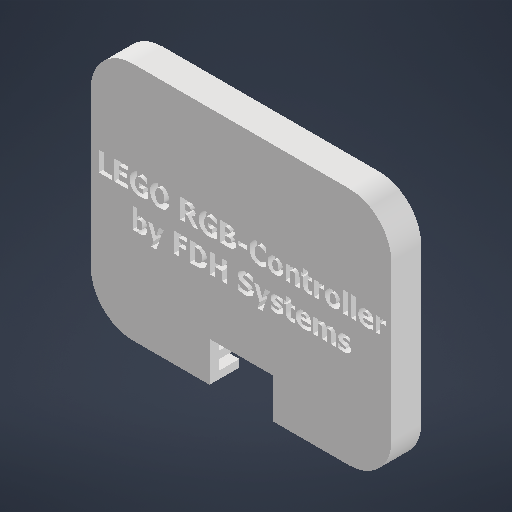
# Autodesk Inventor part: TopShell
Saved by Autodesk Inventor 2026.2 (Build 302298000, 298)
## iProperties
Created: 2026-04-30
Part Number: TopShell
Material: Generic
Document SubType Name: Modeling
Designer: FromDarkHell
Density: 1 g/cm^3
Appearance: Default
Author: FromDarkHell
Autodesk Inventor part; units mm, degrees
ref_plane "YZ Plane" through (0, 0, 0) normal (1, 0, 0) x (0, 1, 0)
ref_plane "XZ Plane" through (0, 0, 0) normal (0, 1, 0) x (-1, 0, 0)
ref_plane "XY Plane" through (0, 0, 0) normal (0, 0, 1) x (1, 0, 0)
sketch "Sketch4" plane through (0, 0, 0) normal (0, 0, 1) x (1, 0, 0)
  arc A0 (29.04, -4) -> (22.04, 3) centre (22.04, -4) ccw projected
  line L0 (29.04, -4) -> (29.04, -35.25) projected
  arc A1 (22.04, -42.25) -> (29.04, -35.25) centre (22.04, -35.25) ccw projected
  line L1 (22.04, -42.25) -> (-21.46, -42.25) projected
  arc A2 (-28.46, -35.25) -> (-21.46, -42.25) centre (-21.46, -35.25) ccw projected
  line L2 (-28.46, -35.25) -> (-28.46, -4) projected
  arc A3 (-21.46, 3) -> (-28.46, -4) centre (-21.46, -4) ccw projected
  line L3 (-21.46, 3) -> (22.04, 3) projected
  line L4 (-26.46, -35.25) -> (-26.46, -4) projected
  arc A4 (-21.46, 1) -> (-26.46, -4) centre (-21.46, -4) ccw projected
  line L5 (-21.46, 1) -> (22.04, 1) projected
  arc A5 (27.04, -4) -> (22.04, 1) centre (22.04, -4) ccw projected
  line L6 (27.04, -4) -> (27.04, -35.25) projected
  arc A6 (22.04, -40.25) -> (27.04, -35.25) centre (22.04, -35.25) ccw projected
  line L7 (22.04, -40.25) -> (-21.46, -40.25) projected
  arc A7 (-26.46, -35.25) -> (-21.46, -40.25) centre (-21.46, -35.25) ccw projected
  line L8 (-29.96, -4) -> (-29.96, -35.25)
  arc A8 (-29.96, -35.25) -> (-21.46, -43.75) centre (-21.46, -35.25) ccw
  line L9 (-21.46, -43.75) -> (22.04, -43.75)
  arc A9 (22.04, -43.75) -> (30.54, -35.25) centre (22.04, -35.25) ccw
  line L10 (30.54, -35.25) -> (30.54, -4)
  arc A10 (30.54, -4) -> (22.04, 4.5) centre (22.04, -4) ccw
  line L11 (22.04, 4.5) -> (-21.46, 4.5)
  arc A11 (-21.46, 4.5) -> (-29.96, -4) centre (-21.46, -4) ccw
  line L12 (-24.96, -4) -> (-24.96, -35.25)
  arc A12 (-24.96, -35.25) -> (-21.46, -38.75) centre (-21.46, -35.25) ccw
  line L13 (-21.46, -38.75) -> (22.04, -38.75)
  arc A13 (22.04, -38.75) -> (25.54, -35.25) centre (22.04, -35.25) ccw
  line L14 (25.54, -35.25) -> (25.54, -4)
  arc A14 (25.54, -4) -> (22.04, -0.5) centre (22.04, -4) ccw
  line L15 (22.04, -0.5) -> (-21.46, -0.5)
  arc A15 (-21.46, -0.5) -> (-24.96, -4) centre (-21.46, -4) ccw
  point P0 (0, 0)
  dimension "d18" = 1.5
  dimension "d19" = 1.5
  constraints: 16 end point, 16 point on circle, 8 centre point, 14 other
  measures "d18" radial gap between concentric circles of A3 A11
  measures "d19" distance between parallel lines of L4 L12
extrude "Extrusion5" add sketch "Sketch4" along normal blind 4
sketch "Sketch5" plane through (0, 0, 4) normal (0, 0, 1) x (1, 0, 0)
  arc A0 (-29.96, -35.25) -> (-21.46, -43.75) centre (-21.46, -35.25) ccw projected
  line L0 (-21.46, -43.75) -> (22.04, -43.75) projected
  arc A1 (22.04, -43.75) -> (30.54, -35.25) centre (22.04, -35.25) ccw projected
  line L1 (30.54, -35.25) -> (30.54, -4) projected
  arc A2 (30.54, -4) -> (22.04, 4.5) centre (22.04, -4) ccw projected
  line L2 (22.04, 4.5) -> (-21.46, 4.5) projected
  arc A3 (-21.46, 4.5) -> (-29.96, -4) centre (-21.46, -4) ccw projected
  line L3 (-29.96, -4) -> (-29.96, -35.25) projected
  line L4 (22.04, -42.25) -> (-21.46, -42.25) projected
  arc A4 (-28.46, -35.25) -> (-21.46, -42.25) centre (-21.46, -35.25) ccw projected
  line L5 (-28.46, -35.25) -> (-28.46, -4) projected
  arc A5 (-21.46, 3) -> (-28.46, -4) centre (-21.46, -4) ccw projected
  line L6 (-21.46, 3) -> (22.04, 3) projected
  arc A6 (29.04, -4) -> (22.04, 3) centre (22.04, -4) ccw projected
  line L7 (29.04, -4) -> (29.04, -35.25) projected
  arc A7 (22.04, -42.25) -> (29.04, -35.25) centre (22.04, -35.25) ccw projected
  point P0 (0, 0)
extrude "Extrusion6" add sketch "Sketch5" along normal blind 2 contours L3 A3 L2 A2 L1 A1 L0 A0 | L4 A4 L5 A5 L6 A6 L7 A7
sketch "Sketch6" plane through (0, 0, 6) normal (0, 0, 1) x (1, 0, 0)
  line L0 (-21.46, -43.75) -> (22.04, -43.75) projected
  arc A0 (22.04, -43.75) -> (30.54, -35.25) centre (22.04, -35.25) ccw projected
  line L1 (30.54, -35.25) -> (30.54, -4) projected
  arc A1 (30.54, -4) -> (22.04, 4.5) centre (22.04, -4) ccw projected
  line L2 (22.04, 4.5) -> (-21.46, 4.5) projected
  arc A2 (-21.46, 4.5) -> (-29.96, -4) centre (-21.46, -4) ccw projected
  line L3 (-29.96, -4) -> (-29.96, -35.25) projected
  arc A3 (-29.96, -35.25) -> (-21.46, -43.75) centre (-21.46, -35.25) ccw projected
  line L4 (-29.96, -19.625) -> (30.54, -19.625) construction
  line L5 (0.29, 4.5) -> (0.29, -43.75) construction
  line L6 (-28.8096, -14.0054) -> (29.3896, -14.0054) construction
  line L7 (29.3896, -14.0054) -> (29.3896, -25.2446) construction
  line L8 (29.3896, -25.2446) -> (-28.8096, -25.2446) construction
  line L9 (-28.8096, -25.2446) -> (-28.8096, -14.0054) construction
  line L10 (-25.7163, -17.8739) -> (-28.3759, -17.8739)
  line L11 (-28.3759, -17.8739) -> (-28.3759, -13.8861)
  line L12 (-28.3759, -13.8861) -> (-27.3741, -13.8861)
  line L13 (-27.3741, -13.8861) -> (-27.3741, -17.1144)
  line L14 (-27.3741, -17.1144) -> (-25.7163, -17.1144)
  line L15 (-25.7163, -17.1144) -> (-25.7163, -17.8739)
  line L16 (-25.2381, -17.8739) -> (-25.2381, -13.8861)
  line L17 (-25.2381, -13.8861) -> (-22.5429, -13.8861)
  line L18 (-22.5429, -13.8861) -> (-22.5429, -14.6455)
  line L19 (-22.5429, -14.6455) -> (-24.2427, -14.6455)
  line L20 (-24.2427, -14.6455) -> (-24.2427, -15.3468)
  line L21 (-24.2427, -15.3468) -> (-22.6754, -15.3468)
  line L22 (-22.6754, -15.3468) -> (-22.6754, -16.1062)
  line L23 (-22.6754, -16.1062) -> (-24.2427, -16.1062)
  line L24 (-24.2427, -16.1062) -> (-24.2427, -17.1144)
  line L25 (-24.2427, -17.1144) -> (-22.5429, -17.1144)
  line L26 (-22.5429, -17.1144) -> (-22.5429, -17.8739)
  line L27 (-22.5429, -17.8739) -> (-25.2381, -17.8739)
  spline S0 degree 2 poles (-18.5357, -17.6477) (-18.7975, -17.7543) (-19.6345, -17.9579) (-20.0416, -17.9579) knots 0 0 0 1 2 2 2
  spline S1 degree 2 poles (-20.0416, -17.9579) (-20.982, -17.9579) (-22.0969, -16.8721) (-22.0969, -15.8767) knots 0 0 0 1 2 2 2
  spline S2 degree 2 poles (-22.0969, -15.8767) (-22.0969, -14.9396) (-20.982, -13.8085) (-20.0126, -13.8085) knots 0 0 0 1 2 2 2
  spline S3 degree 2 poles (-20.0126, -13.8085) (-19.5117, -13.8085) (-18.8847, -13.9992) (-18.5519, -14.1608) knots 0 0 0 1 2 2 2
  line L28 (-18.5519, -14.1608) -> (-18.5519, -15.0979)
  line L29 (-18.5519, -15.0979) -> (-18.6424, -15.0979)
  spline S4 degree 2 poles (-18.6424, -15.0979) (-18.7134, -15.043) (-18.9849, -14.8329) (-19.1142, -14.7618) knots 0 0 0 1 2 2 2
  spline S5 degree 2 poles (-19.1142, -14.7618) (-19.2628, -14.6746) (-19.6571, -14.5518) (-19.8768, -14.5518) knots 0 0 0 1 2 2 2
  spline S6 degree 2 poles (-19.8768, -14.5518) (-20.1321, -14.5518) (-20.5555, -14.7134) (-20.7203, -14.8782) knots 0 0 0 1 2 2 2
  spline S7 degree 2 poles (-20.7203, -14.8782) (-20.8786, -15.0398) (-21.0628, -15.5342) (-21.0628, -15.8606) knots 0 0 0 1 2 2 2
  spline S8 degree 2 poles (-21.0628, -15.8606) (-21.0628, -16.5586) (-20.3616, -17.2243) (-19.7573, -17.2243) knots 0 0 0 1 2 2 2
  spline S9 degree 2 poles (-19.7573, -17.2243) (-19.7023, -17.2243) (-19.5601, -17.2179) (-19.5052, -17.2146) knots 0 0 0 1 2 2 2
  line L30 (-19.5052, -17.2146) -> (-19.5052, -16.4293)
  line L31 (-19.5052, -16.4293) -> (-20.2775, -16.4293)
  line L32 (-20.2775, -16.4293) -> (-20.2775, -15.6828)
  line L33 (-20.2775, -15.6828) -> (-18.5357, -15.6828)
  line L34 (-18.5357, -15.6828) -> (-18.5357, -17.6477)
  spline S10 degree 2 poles (-14.1504, -15.88) (-14.1504, -16.8495) (-15.1845, -17.9579) (-16.0829, -17.9579) knots 0 0 0 1 2 2 2
  spline S11 degree 2 poles (-16.0829, -17.9579) (-16.9845, -17.9579) (-18.0122, -16.8365) (-18.0122, -15.88) knots 0 0 0 1 2 2 2
  spline S12 degree 2 poles (-18.0122, -15.88) (-18.0122, -14.9202) (-16.9845, -13.8021) (-16.0829, -13.8021) knots 0 0 0 1 2 2 2
  spline S13 degree 2 poles (-16.0829, -13.8021) (-15.1845, -13.8021) (-14.1504, -14.9137) (-14.1504, -15.88) knots 0 0 0 1 2 2 2
  spline S14 degree 2 poles (-15.1845, -15.88) (-15.1845, -15.5213) (-15.33, -15.0204) (-15.456, -14.862) knots 0 0 0 1 2 2 2
  spline S15 degree 2 poles (-15.456, -14.862) (-15.582, -14.6972) (-15.9052, -14.555) (-16.0797, -14.555) knots 0 0 0 1 2 2 2
  spline S16 degree 2 poles (-16.0797, -14.555) (-16.2639, -14.555) (-16.5644, -14.6875) (-16.7034, -14.8556) knots 0 0 0 1 2 2 2
  spline S17 degree 2 poles (-16.7034, -14.8556) (-16.8262, -15.0107) (-16.9781, -15.5245) (-16.9781, -15.88) knots 0 0 0 1 2 2 2
  spline S18 degree 2 poles (-16.9781, -15.88) (-16.9781, -16.2484) (-16.8327, -16.7331) (-16.7066, -16.8979) knots 0 0 0 1 2 2 2
  spline S19 degree 2 poles (-16.7066, -16.8979) (-16.5806, -17.0627) (-16.2542, -17.2049) (-16.0797, -17.2049) knots 0 0 0 1 2 2 2
  spline S20 degree 2 poles (-16.0797, -17.2049) (-15.902, -17.2049) (-15.5723, -17.053) (-15.4528, -16.8915) knots 0 0 0 1 2 2 2
  spline S21 degree 2 poles (-15.4528, -16.8915) (-15.3235, -16.717) (-15.1845, -16.2548) (-15.1845, -15.88) knots 0 0 0 1 2 2 2
  line L35 (-8.2657, -17.8739) -> (-9.484, -17.8739)
  line L36 (-9.484, -17.8739) -> (-10.5924, -16.41)
  line L37 (-10.5924, -16.41) -> (-10.9544, -16.41)
  line L38 (-10.9544, -16.41) -> (-10.9544, -17.8739)
  line L39 (-10.9544, -17.8739) -> (-11.9497, -17.8739)
  line L40 (-11.9497, -17.8739) -> (-11.9497, -13.8861)
  line L41 (-11.9497, -13.8861) -> (-10.3468, -13.8861)
  spline S22 degree 2 poles (-10.3468, -13.8861) (-10.014, -13.8861) (-9.5228, -13.9701) (-9.3127, -14.0994) knots 0 0 0 1 2 2 2
  spline S23 degree 2 poles (-9.3127, -14.0994) (-9.0994, -14.2351) (-8.8474, -14.6584) (-8.8474, -14.9816) knots 0 0 0 1 2 2 2
  spline S24 degree 2 poles (-8.8474, -14.9816) (-8.8474, -15.4372) (-9.261, -16.0092) (-9.6068, -16.1773) knots 0 0 0 1 2 2 2
  line L42 (-9.6068, -16.1773) -> (-8.2657, -17.8739)
  spline S25 degree 2 poles (-9.875, -15.1076) (-9.875, -14.9557) (-9.9913, -14.7392) (-10.1238, -14.6811) knots 0 0 0 1 2 2 2
  spline S26 degree 2 poles (-10.1238, -14.6811) (-10.2176, -14.6423) (-10.447, -14.6197) (-10.6183, -14.6197) knots 0 0 0 1 2 2 2
  line L43 (-10.6183, -14.6197) -> (-10.9544, -14.6197)
  line L44 (-10.9544, -14.6197) -> (-10.9544, -15.6925)
  line L45 (-10.9544, -15.6925) -> (-10.6668, -15.6925)
  spline S27 degree 2 poles (-10.6668, -15.6925) (-10.4599, -15.6925) (-10.1659, -15.6408) (-10.0657, -15.56) knots 0 0 0 1 2 2 2
  spline S28 degree 2 poles (-10.0657, -15.56) (-9.9687, -15.4825) (-9.875, -15.2757) (-9.875, -15.1076) knots 0 0 0 1 2 2 2
  spline S29 degree 2 poles (-4.6398, -17.6477) (-4.9016, -17.7543) (-5.7386, -17.9579) (-6.1457, -17.9579) knots 0 0 0 1 2 2 2
  spline S30 degree 2 poles (-6.1457, -17.9579) (-7.0861, -17.9579) (-8.201, -16.8721) (-8.201, -15.8767) knots 0 0 0 1 2 2 2
  spline S31 degree 2 poles (-8.201, -15.8767) (-8.201, -14.9396) (-7.0861, -13.8085) (-6.1167, -13.8085) knots 0 0 0 1 2 2 2
  spline S32 degree 2 poles (-6.1167, -13.8085) (-5.6158, -13.8085) (-4.9888, -13.9992) (-4.656, -14.1608) knots 0 0 0 1 2 2 2
  line L46 (-4.656, -14.1608) -> (-4.656, -15.0979)
  line L47 (-4.656, -15.0979) -> (-4.7465, -15.0979)
  spline S33 degree 2 poles (-4.7465, -15.0979) (-4.8176, -15.043) (-5.089, -14.8329) (-5.2183, -14.7618) knots 0 0 0 1 2 2 2
  spline S34 degree 2 poles (-5.2183, -14.7618) (-5.3669, -14.6746) (-5.7612, -14.5518) (-5.9809, -14.5518) knots 0 0 0 1 2 2 2
  spline S35 degree 2 poles (-5.9809, -14.5518) (-6.2362, -14.5518) (-6.6596, -14.7134) (-6.8244, -14.8782) knots 0 0 0 1 2 2 2
  spline S36 degree 2 poles (-6.8244, -14.8782) (-6.9827, -15.0398) (-7.1669, -15.5342) (-7.1669, -15.8606) knots 0 0 0 1 2 2 2
  spline S37 degree 2 poles (-7.1669, -15.8606) (-7.1669, -16.5586) (-6.4657, -17.2243) (-5.8614, -17.2243) knots 0 0 0 1 2 2 2
  spline S38 degree 2 poles (-5.8614, -17.2243) (-5.8064, -17.2243) (-5.6642, -17.2179) (-5.6093, -17.2146) knots 0 0 0 1 2 2 2
  line L48 (-5.6093, -17.2146) -> (-5.6093, -16.4293)
  line L49 (-5.6093, -16.4293) -> (-6.3816, -16.4293)
  line L50 (-6.3816, -16.4293) -> (-6.3816, -15.6828)
  line L51 (-6.3816, -15.6828) -> (-4.6398, -15.6828)
  line L52 (-4.6398, -15.6828) -> (-4.6398, -17.6477)
  spline S39 degree 2 poles (-0.6973, -16.6523) (-0.6973, -16.9496) (-0.9235, -17.3988) (-1.1109, -17.5475) knots 0 0 0 1 2 2 2
  spline S40 degree 2 poles (-1.1109, -17.5475) (-1.3371, -17.7252) (-1.8736, -17.8739) (-2.2904, -17.8739) knots 0 0 0 1 2 2 2
  line L53 (-2.2904, -17.8739) -> (-3.8836, -17.8739)
  line L54 (-3.8836, -17.8739) -> (-3.8836, -13.8861)
  line L55 (-3.8836, -13.8861) -> (-2.4779, -13.8861)
  spline S41 degree 2 poles (-2.4779, -13.8861) (-2.0384, -13.8861) (-1.5859, -13.9539) (-1.3888, -14.0606) knots 0 0 0 1 2 2 2
  spline S42 degree 2 poles (-1.3888, -14.0606) (-1.1723, -14.1737) (-0.9622, -14.5615) (-0.9622, -14.8135) knots 0 0 0 1 2 2 2
  spline S43 degree 2 poles (-0.9622, -14.8135) (-0.9622, -15.1044) (-1.2531, -15.56) (-1.5116, -15.6667) knots 0 0 0 1 2 2 2
  line L56 (-1.5116, -15.6667) -> (-1.5116, -15.6861)
  spline S44 degree 2 poles (-1.5116, -15.6861) (-1.14, -15.7636) (-0.6973, -16.2451) (-0.6973, -16.6523) knots 0 0 0 1 2 2 2
  spline S45 degree 2 poles (-1.7314, -16.6362) (-1.7314, -16.4487) (-1.88, -16.2387) (-2.0287, -16.1837) knots 0 0 0 1 2 2 2
  spline S46 degree 2 poles (-2.0287, -16.1837) (-2.1192, -16.1482) (-2.4391, -16.1417) (-2.7041, -16.1417) knots 0 0 0 1 2 2 2
  line L57 (-2.7041, -16.1417) -> (-2.8883, -16.1417)
  line L58 (-2.8883, -16.1417) -> (-2.8883, -17.1468)
  line L59 (-2.8883, -17.1468) -> (-2.8333, -17.1468)
  spline S47 degree 2 poles (-2.8333, -17.1468) (-2.4456, -17.1468) (-2.1482, -17.1371) (-1.9931, -17.0692) knots 0 0 0 1 2 2 2
  spline S48 degree 2 poles (-1.9931, -17.0692) (-1.8574, -17.0078) (-1.7314, -16.7816) (-1.7314, -16.6362) knots 0 0 0 1 2 2 2
  spline S49 degree 2 poles (-1.9802, -15.0107) (-1.9802, -14.9137) (-2.0804, -14.7101) (-2.1838, -14.6649) knots 0 0 0 1 2 2 2
  spline S50 degree 2 poles (-2.1838, -14.6649) (-2.2807, -14.6197) (-2.5522, -14.6132) (-2.8204, -14.6132) knots 0 0 0 1 2 2 2
  line L60 (-2.8204, -14.6132) -> (-2.8883, -14.6132)
  line L61 (-2.8883, -14.6132) -> (-2.8883, -15.4599)
  line L62 (-2.8883, -15.4599) -> (-2.7623, -15.4599)
  spline S51 degree 2 poles (-2.7623, -15.4599) (-2.507, -15.4599) (-2.3001, -15.4502) (-2.1903, -15.3985) knots 0 0 0 1 2 2 2
  spline S52 degree 2 poles (-2.1903, -15.3985) (-2.0707, -15.3403) (-1.9802, -15.1432) (-1.9802, -15.0107) knots 0 0 0 1 2 2 2
  line L63 (1.5326, -16.4843) -> (-0.2416, -16.4843)
  line L64 (-0.2416, -16.4843) -> (-0.2416, -15.741)
  line L65 (-0.2416, -15.741) -> (1.5326, -15.741)
  line L66 (1.5326, -15.741) -> (1.5326, -16.4843)
  spline S53 degree 2 poles (3.9627, -17.9514) (3.0643, -17.9514) (2.0108, -16.8656) (2.0108, -15.8832) knots 0 0 0 1 2 2 2
  spline S54 degree 2 poles (2.0108, -15.8832) (2.0108, -14.9363) (3.0676, -13.8085) (3.966, -13.8085) knots 0 0 0 1 2 2 2
  spline S55 degree 2 poles (3.966, -13.8085) (4.2019, -13.8085) (4.5832, -13.8635) (4.7577, -13.9087) knots 0 0 0 1 2 2 2
  spline S56 degree 2 poles (4.7577, -13.9087) (4.8934, -13.9507) (5.2133, -14.0897) (5.3135, -14.1414) knots 0 0 0 1 2 2 2
  line L67 (5.3135, -14.1414) -> (5.3135, -15.0915)
  line L68 (5.3135, -15.0915) -> (5.2133, -15.0915)
  spline S57 degree 2 poles (5.2133, -15.0915) (5.139, -15.0268) (4.9193, -14.8459) (4.7803, -14.7618) knots 0 0 0 1 2 2 2
  spline S58 degree 2 poles (4.7803, -14.7618) (4.6414, -14.6746) (4.3085, -14.555) (4.1243, -14.555) knots 0 0 0 1 2 2 2
  spline S59 degree 2 poles (4.1243, -14.555) (3.9078, -14.555) (3.5491, -14.6907) (3.3843, -14.862) knots 0 0 0 1 2 2 2
  spline S60 degree 2 poles (3.3843, -14.862) (3.2356, -15.0139) (3.0449, -15.5342) (3.0449, -15.8864) knots 0 0 0 1 2 2 2
  spline S61 degree 2 poles (3.0449, -15.8864) (3.0449, -16.2581) (3.2421, -16.7654) (3.4037, -16.9206) knots 0 0 0 1 2 2 2
  spline S62 degree 2 poles (3.4037, -16.9206) (3.5588, -17.0724) (3.9401, -17.2049) (4.1308, -17.2049) knots 0 0 0 1 2 2 2
  spline S63 degree 2 poles (4.1308, -17.2049) (4.3279, -17.2049) (4.6866, -17.0724) (4.8094, -16.9916) knots 0 0 0 1 2 2 2
  spline S64 degree 2 poles (4.8094, -16.9916) (4.9451, -16.9109) (5.1487, -16.7396) (5.223, -16.6717) knots 0 0 0 1 2 2 2
  line L69 (5.223, -16.6717) -> (5.3135, -16.6717)
  line L70 (5.3135, -16.6717) -> (5.3135, -17.6089)
  spline S65 degree 2 poles (5.3135, -17.6089) (5.2037, -17.6606) (4.916, -17.7899) (4.7609, -17.8351) knots 0 0 0 1 2 2 2
  spline S66 degree 2 poles (4.7609, -17.8351) (4.5735, -17.8933) (4.2471, -17.9514) (3.9627, -17.9514) knots 0 0 0 1 2 2 2
  spline S67 degree 2 poles (8.7358, -16.3712) (8.7358, -17.1144) (7.9247, -17.9676) (7.1846, -17.9676) knots 0 0 0 1 2 2 2
  spline S68 degree 2 poles (7.1846, -17.9676) (6.4478, -17.9676) (5.6302, -17.1144) (5.6302, -16.3712) knots 0 0 0 1 2 2 2
  spline S69 degree 2 poles (5.6302, -16.3712) (5.6302, -15.6214) (6.4478, -14.7715) (7.1846, -14.7715) knots 0 0 0 1 2 2 2
  spline S70 degree 2 poles (7.1846, -14.7715) (7.9214, -14.7715) (8.7358, -15.6247) (8.7358, -16.3712) knots 0 0 0 1 2 2 2
  spline S71 degree 2 poles (7.776, -16.3776) (7.776, -16.1094) (7.6888, -15.7507) (7.6112, -15.6441) knots 0 0 0 1 2 2 2
  spline S72 degree 2 poles (7.6112, -15.6441) (7.5272, -15.531) (7.3171, -15.4437) (7.1846, -15.4437) knots 0 0 0 1 2 2 2
  spline S73 degree 2 poles (7.1846, -15.4437) (7.0554, -15.4437) (6.8518, -15.5213) (6.7678, -15.6311) knots 0 0 0 1 2 2 2
  spline S74 degree 2 poles (6.7678, -15.6311) (6.687, -15.7346) (6.59, -16.0997) (6.59, -16.3776) knots 0 0 0 1 2 2 2
  spline S75 degree 2 poles (6.59, -16.3776) (6.59, -16.6523) (6.6805, -16.9916) (6.7548, -17.0951) knots 0 0 0 1 2 2 2
  spline S76 degree 2 poles (6.7548, -17.0951) (6.8292, -17.1985) (7.0554, -17.2954) (7.1911, -17.2954) knots 0 0 0 1 2 2 2
  spline S77 degree 2 poles (7.1911, -17.2954) (7.3042, -17.2954) (7.5369, -17.1985) (7.608, -17.1015) knots 0 0 0 1 2 2 2
  spline S78 degree 2 poles (7.608, -17.1015) (7.6888, -16.9884) (7.776, -16.662) (7.776, -16.3776) knots 0 0 0 1 2 2 2
  line L71 (12.0482, -17.8739) -> (11.1046, -17.8739)
  line L72 (11.1046, -17.8739) -> (11.1046, -16.3841)
  spline S79 degree 2 poles (11.1046, -16.3841) (11.1046, -16.1999) (11.0755, -15.838) (11.0367, -15.7539) knots 0 0 0 1 2 2 2
  spline S80 degree 2 poles (11.0367, -15.7539) (10.9882, -15.6505) (10.8073, -15.5633) (10.6521, -15.5633) knots 0 0 0 1 2 2 2
  spline S81 degree 2 poles (10.6521, -15.5633) (10.539, -15.5633) (10.3031, -15.6505) (10.1706, -15.7442) knots 0 0 0 1 2 2 2
  line L73 (10.1706, -15.7442) -> (10.1706, -17.8739)
  line L74 (10.1706, -17.8739) -> (9.2335, -17.8739)
  line L75 (9.2335, -17.8739) -> (9.2335, -14.8653)
  line L76 (9.2335, -14.8653) -> (10.1706, -14.8653)
  line L77 (10.1706, -14.8653) -> (10.1706, -15.1981)
  spline S82 degree 2 poles (10.1706, -15.1981) (10.4001, -15.0042) (10.8363, -14.7845) (11.1013, -14.7845) knots 0 0 0 1 2 2 2
  spline S83 degree 2 poles (11.1013, -14.7845) (11.5602, -14.7845) (12.0482, -15.3662) (12.0482, -15.9155) knots 0 0 0 1 2 2 2
  line L78 (12.0482, -15.9155) -> (12.0482, -17.8739)
  spline S84 degree 2 poles (13.8934, -17.932) (13.3214, -17.932) (12.7979, -17.4602) (12.7979, -16.9238) knots 0 0 0 1 2 2 2
  line L79 (12.7979, -16.9238) -> (12.7979, -15.518)
  line L80 (12.7979, -15.518) -> (12.4392, -15.518)
  line L81 (12.4392, -15.518) -> (12.4392, -14.8653)
  line L82 (12.4392, -14.8653) -> (12.7979, -14.8653)
  line L83 (12.7979, -14.8653) -> (12.7979, -14.0056)
  line L84 (12.7979, -14.0056) -> (13.7351, -14.0056)
  line L85 (13.7351, -14.0056) -> (13.7351, -14.8653)
  line L86 (13.7351, -14.8653) -> (14.6399, -14.8653)
  line L87 (14.6399, -14.8653) -> (14.6399, -15.518)
  line L88 (14.6399, -15.518) -> (13.7351, -15.518)
  line L89 (13.7351, -15.518) -> (13.7351, -16.5877)
  spline S85 degree 2 poles (13.7351, -16.5877) (13.7351, -16.746) (13.7416, -16.982) (13.7803, -17.0757) knots 0 0 0 1 2 2 2
  spline S86 degree 2 poles (13.7803, -17.0757) (13.8191, -17.1694) (14.0098, -17.2793) (14.1907, -17.2793) knots 0 0 0 1 2 2 2
  spline S87 degree 2 poles (14.1907, -17.2793) (14.2683, -17.2793) (14.5107, -17.2146) (14.5591, -17.1888) knots 0 0 0 1 2 2 2
  line L90 (14.5591, -17.1888) -> (14.6399, -17.1888)
  line L91 (14.6399, -17.1888) -> (14.6399, -17.848)
  spline S88 degree 2 poles (14.6399, -17.848) (14.4881, -17.8868) (14.1455, -17.932) (13.8934, -17.932) knots 0 0 0 1 2 2 2
  line L92 (17.041, -15.7539) -> (16.9635, -15.7539)
  spline S89 degree 2 poles (16.9635, -15.7539) (16.9085, -15.7346) (16.7049, -15.7152) (16.5821, -15.7152) knots 0 0 0 1 2 2 2
  spline S90 degree 2 poles (16.5821, -15.7152) (16.4367, -15.7152) (16.1103, -15.8024) (15.9584, -15.8606) knots 0 0 0 1 2 2 2
  line L93 (15.9584, -15.8606) -> (15.9584, -17.8739)
  line L94 (15.9584, -17.8739) -> (15.0213, -17.8739)
  line L95 (15.0213, -17.8739) -> (15.0213, -14.8653)
  line L96 (15.0213, -14.8653) -> (15.9584, -14.8653)
  line L97 (15.9584, -14.8653) -> (15.9584, -15.2983)
  spline S91 degree 2 poles (15.9584, -15.2983) (16.0231, -15.2401) (16.2493, -15.0591) (16.343, -15.0042) knots 0 0 0 1 2 2 2
  spline S92 degree 2 poles (16.343, -15.0042) (16.4464, -14.9428) (16.7179, -14.8556) (16.8374, -14.8556) knots 0 0 0 1 2 2 2
  spline S93 degree 2 poles (16.8374, -14.8556) (16.8827, -14.8556) (16.9958, -14.862) (17.041, -14.8653) knots 0 0 0 1 2 2 2
  line L98 (17.041, -14.8653) -> (17.041, -15.7539)
  spline S94 degree 2 poles (20.2856, -16.3712) (20.2856, -17.1144) (19.4744, -17.9676) (18.7344, -17.9676) knots 0 0 0 1 2 2 2
  spline S95 degree 2 poles (18.7344, -17.9676) (17.9976, -17.9676) (17.18, -17.1144) (17.18, -16.3712) knots 0 0 0 1 2 2 2
  spline S96 degree 2 poles (17.18, -16.3712) (17.18, -15.6214) (17.9976, -14.7715) (18.7344, -14.7715) knots 0 0 0 1 2 2 2
  spline S97 degree 2 poles (18.7344, -14.7715) (19.4712, -14.7715) (20.2856, -15.6247) (20.2856, -16.3712) knots 0 0 0 1 2 2 2
  spline S98 degree 2 poles (19.3258, -16.3776) (19.3258, -16.1094) (19.2385, -15.7507) (19.161, -15.6441) knots 0 0 0 1 2 2 2
  spline S99 degree 2 poles (19.161, -15.6441) (19.0769, -15.531) (18.8669, -15.4437) (18.7344, -15.4437) knots 0 0 0 1 2 2 2
  spline S100 degree 2 poles (18.7344, -15.4437) (18.6051, -15.4437) (18.4015, -15.5213) (18.3175, -15.6311) knots 0 0 0 1 2 2 2
  spline S101 degree 2 poles (18.3175, -15.6311) (18.2367, -15.7346) (18.1398, -16.0997) (18.1398, -16.3776) knots 0 0 0 1 2 2 2
  spline S102 degree 2 poles (18.1398, -16.3776) (18.1398, -16.6523) (18.2303, -16.9916) (18.3046, -17.0951) knots 0 0 0 1 2 2 2
  spline S103 degree 2 poles (18.3046, -17.0951) (18.3789, -17.1985) (18.6051, -17.2954) (18.7408, -17.2954) knots 0 0 0 1 2 2 2
  spline S104 degree 2 poles (18.7408, -17.2954) (18.854, -17.2954) (19.0866, -17.1985) (19.1577, -17.1015) knots 0 0 0 1 2 2 2
  spline S105 degree 2 poles (19.1577, -17.1015) (19.2385, -16.9884) (19.3258, -16.662) (19.3258, -16.3776) knots 0 0 0 1 2 2 2
  line L99 (21.7204, -17.8739) -> (20.7832, -17.8739)
  line L100 (20.7832, -17.8739) -> (20.7832, -13.7083)
  line L101 (20.7832, -13.7083) -> (21.7204, -13.7083)
  line L102 (21.7204, -13.7083) -> (21.7204, -17.8739)
  line L103 (23.375, -17.8739) -> (22.4378, -17.8739)
  line L104 (22.4378, -17.8739) -> (22.4378, -13.7083)
  line L105 (22.4378, -13.7083) -> (23.375, -13.7083)
  line L106 (23.375, -13.7083) -> (23.375, -17.8739)
  spline S106 degree 2 poles (25.6339, -17.9547) (24.7807, -17.9547) (23.8726, -17.1403) (23.8726, -16.3873) knots 0 0 0 1 2 2 2
  spline S107 degree 2 poles (23.8726, -16.3873) (23.8726, -15.6505) (24.7193, -14.7715) (25.482, -14.7715) knots 0 0 0 1 2 2 2
  spline S108 degree 2 poles (25.482, -14.7715) (26.1703, -14.7715) (26.8683, -15.518) (26.8683, -16.2096) knots 0 0 0 1 2 2 2
  line L107 (26.8683, -16.2096) -> (26.8683, -16.5489)
  line L108 (26.8683, -16.5489) -> (24.8098, -16.5489)
  spline S109 degree 2 poles (24.8098, -16.5489) (24.8227, -16.759) (24.9746, -17.0369) (25.0974, -17.1209) knots 0 0 0 1 2 2 2
  spline S110 degree 2 poles (25.0974, -17.1209) (25.217, -17.2049) (25.5401, -17.276) (25.7308, -17.276) knots 0 0 0 1 2 2 2
  spline S111 degree 2 poles (25.7308, -17.276) (25.8924, -17.276) (26.2091, -17.2049) (26.3416, -17.1435) knots 0 0 0 1 2 2 2
  spline S112 degree 2 poles (26.3416, -17.1435) (26.4579, -17.0951) (26.6518, -16.9755) (26.7132, -16.9302) knots 0 0 0 1 2 2 2
  line L109 (26.7132, -16.9302) -> (26.8134, -16.9302)
  line L110 (26.8134, -16.9302) -> (26.8134, -17.7058)
  spline S113 degree 2 poles (26.8134, -17.7058) (26.6971, -17.7511) (26.5096, -17.8286) (26.3416, -17.8674) knots 0 0 0 1 2 2 2
  spline S114 degree 2 poles (26.3416, -17.8674) (26.1897, -17.9094) (25.8665, -17.9547) (25.6339, -17.9547) knots 0 0 0 1 2 2 2
  spline S115 degree 2 poles (25.9441, -15.9834) (25.9376, -15.6861) (25.6759, -15.3726) (25.4076, -15.3726) knots 0 0 0 1 2 2 2
  spline S116 degree 2 poles (25.4076, -15.3726) (25.133, -15.3726) (24.8227, -15.7022) (24.8066, -15.9834) knots 0 0 0 1 2 2 2
  line L111 (24.8066, -15.9834) -> (25.9441, -15.9834)
  line L112 (29.3696, -15.7539) -> (29.292, -15.7539)
  spline S117 degree 2 poles (29.292, -15.7539) (29.2371, -15.7346) (29.0335, -15.7152) (28.9107, -15.7152) knots 0 0 0 1 2 2 2
  spline S118 degree 2 poles (28.9107, -15.7152) (28.7653, -15.7152) (28.4389, -15.8024) (28.287, -15.8606) knots 0 0 0 1 2 2 2
  line L113 (28.287, -15.8606) -> (28.287, -17.8739)
  line L114 (28.287, -17.8739) -> (27.3498, -17.8739)
  line L115 (27.3498, -17.8739) -> (27.3498, -14.8653)
  line L116 (27.3498, -14.8653) -> (28.287, -14.8653)
  line L117 (28.287, -14.8653) -> (28.287, -15.2983)
  spline S119 degree 2 poles (28.287, -15.2983) (28.3516, -15.2401) (28.5778, -15.0591) (28.6716, -15.0042) knots 0 0 0 1 2 2 2
  spline S120 degree 2 poles (28.6716, -15.0042) (28.775, -14.9428) (29.0464, -14.8556) (29.166, -14.8556) knots 0 0 0 1 2 2 2
  spline S121 degree 2 poles (29.166, -14.8556) (29.2112, -14.8556) (29.3244, -14.862) (29.3696, -14.8653) knots 0 0 0 1 2 2 2
  line L118 (29.3696, -14.8653) -> (29.3696, -15.7539)
  spline S122 degree 2 poles (-18.6052, -22.895) (-18.6052, -23.6124) (-19.3323, -24.4979) (-19.872, -24.4979) knots 0 0 0 1 2 2 2
  spline S123 degree 2 poles (-19.872, -24.4979) (-20.095, -24.4979) (-20.4278, -24.3977) (-20.6152, -24.291) knots 0 0 0 1 2 2 2
  line L119 (-20.6152, -24.291) -> (-20.654, -24.4397)
  line L120 (-20.654, -24.4397) -> (-21.5524, -24.4397)
  line L121 (-21.5524, -24.4397) -> (-21.5524, -20.2741)
  line L122 (-21.5524, -20.2741) -> (-20.6152, -20.2741)
  line L123 (-20.6152, -20.2741) -> (-20.6152, -21.7478)
  spline S124 degree 2 poles (-20.6152, -21.7478) (-20.4084, -21.57) (-19.9819, -21.3503) (-19.7007, -21.3503) knots 0 0 0 1 2 2 2
  spline S125 degree 2 poles (-19.7007, -21.3503) (-19.174, -21.3503) (-18.6052, -22.1679) (-18.6052, -22.895) knots 0 0 0 1 2 2 2
  spline S126 degree 2 poles (-19.565, -22.9144) (-19.565, -22.4652) (-19.8364, -22.0806) (-20.1208, -22.0806) knots 0 0 0 1 2 2 2
  spline S127 degree 2 poles (-20.1208, -22.0806) (-20.2468, -22.0806) (-20.4957, -22.1614) (-20.6152, -22.2422) knots 0 0 0 1 2 2 2
  line L124 (-20.6152, -22.2422) -> (-20.6152, -23.7481)
  spline S128 degree 2 poles (-20.6152, -23.7481) (-20.5215, -23.7869) (-20.3309, -23.8128) (-20.2371, -23.8128) knots 0 0 0 1 2 2 2
  spline S129 degree 2 poles (-20.2371, -23.8128) (-19.8978, -23.8128) (-19.565, -23.3636) (-19.565, -22.9144) knots 0 0 0 1 2 2 2
  line L125 (-15.2831, -21.4311) -> (-16.7987, -25.5417)
  line L126 (-16.7987, -25.5417) -> (-17.807, -25.5417)
  line L127 (-17.807, -25.5417) -> (-17.3513, -24.3654)
  line L128 (-17.3513, -24.3654) -> (-18.4533, -21.4311)
  line L129 (-18.4533, -21.4311) -> (-17.4709, -21.4311)
  line L130 (-17.4709, -21.4311) -> (-16.8375, -23.3183)
  line L131 (-16.8375, -23.3183) -> (-16.2461, -21.4311)
  line L132 (-16.2461, -21.4311) -> (-15.2831, -21.4311)
  line L133 (-10.6005, -21.2113) -> (-12.2745, -21.2113)
  line L134 (-12.2745, -21.2113) -> (-12.2745, -21.9643)
  line L135 (-12.2745, -21.9643) -> (-10.733, -21.9643)
  line L136 (-10.733, -21.9643) -> (-10.733, -22.7237)
  line L137 (-10.733, -22.7237) -> (-12.2745, -22.7237)
  line L138 (-12.2745, -22.7237) -> (-12.2745, -24.4397)
  line L139 (-12.2745, -24.4397) -> (-13.2698, -24.4397)
  line L140 (-13.2698, -24.4397) -> (-13.2698, -20.4519)
  line L141 (-13.2698, -20.4519) -> (-10.6005, -20.4519)
  line L142 (-10.6005, -20.4519) -> (-10.6005, -21.2113)
  spline S130 degree 2 poles (-6.5255, -22.449) (-6.5255, -23.0081) (-7.0134, -23.8871) (-7.3851, -24.123) knots 0 0 0 1 2 2 2
  spline S131 degree 2 poles (-7.3851, -24.123) (-7.6953, -24.3233) (-8.4256, -24.4397) (-8.836, -24.4397) knots 0 0 0 1 2 2 2
  line L143 (-8.836, -24.4397) -> (-10.0834, -24.4397)
  line L144 (-10.0834, -24.4397) -> (-10.0834, -20.4519)
  line L145 (-10.0834, -20.4519) -> (-8.849, -20.4519)
  spline S132 degree 2 poles (-8.849, -20.4519) (-8.4289, -20.4519) (-7.6953, -20.5585) (-7.3721, -20.7653) knots 0 0 0 1 2 2 2
  spline S133 degree 2 poles (-7.3721, -20.7653) (-6.9811, -21.0174) (-6.5255, -21.8706) (-6.5255, -22.449) knots 0 0 0 1 2 2 2
  spline S134 degree 2 poles (-7.5531, -22.4426) (-7.5531, -22.0483) (-7.8246, -21.486) (-8.1025, -21.3276) knots 0 0 0 1 2 2 2
  spline S135 degree 2 poles (-8.1025, -21.3276) (-8.3061, -21.2178) (-8.752, -21.1952) (-9.0623, -21.1952) knots 0 0 0 1 2 2 2
  line L146 (-9.0623, -21.1952) -> (-9.0817, -21.1952)
  line L147 (-9.0817, -21.1952) -> (-9.0817, -23.6932)
  line L148 (-9.0817, -23.6932) -> (-9.0623, -23.6932)
  spline S136 degree 2 poles (-9.0623, -23.6932) (-8.7262, -23.6932) (-8.2641, -23.6706) (-8.054, -23.5381) knots 0 0 0 1 2 2 2
  spline S137 degree 2 poles (-8.054, -23.5381) (-7.8084, -23.3829) (-7.5531, -22.8368) (-7.5531, -22.4426) knots 0 0 0 1 2 2 2
  line L149 (-2.5667, -24.4397) -> (-3.5685, -24.4397)
  line L150 (-3.5685, -24.4397) -> (-3.5685, -22.672)
  line L151 (-3.5685, -22.672) -> (-4.929, -22.672)
  line L152 (-4.929, -22.672) -> (-4.929, -24.4397)
  line L153 (-4.929, -24.4397) -> (-5.9308, -24.4397)
  line L154 (-5.9308, -24.4397) -> (-5.9308, -20.4519)
  line L155 (-5.9308, -20.4519) -> (-4.929, -20.4519)
  line L156 (-4.929, -20.4519) -> (-4.929, -21.9126)
  line L157 (-4.929, -21.9126) -> (-3.5685, -21.9126)
  line L158 (-3.5685, -21.9126) -> (-3.5685, -20.4519)
  line L159 (-3.5685, -20.4519) -> (-2.5667, -20.4519)
  line L160 (-2.5667, -20.4519) -> (-2.5667, -24.4397)
  spline S138 degree 2 poles (1.0979, -24.5108) (0.639, -24.5108) (-0.0525, -24.333) (-0.3499, -24.2038) knots 0 0 0 1 2 2 2
  line L161 (-0.3499, -24.2038) -> (-0.3499, -23.2537)
  line L162 (-0.3499, -23.2537) -> (-0.2594, -23.2537)
  spline S139 degree 2 poles (-0.2594, -23.2537) (0.0412, -23.509) (0.7618, -23.7837) (1.1011, -23.7837) knots 0 0 0 1 2 2 2
  spline S140 degree 2 poles (1.1011, -23.7837) (1.1884, -23.7837) (1.4695, -23.7449) (1.5536, -23.7061) knots 0 0 0 1 2 2 2
  spline S141 degree 2 poles (1.5536, -23.7061) (1.657, -23.6609) (1.8024, -23.4961) (1.8024, -23.3636) knots 0 0 0 1 2 2 2
  spline S142 degree 2 poles (1.8024, -23.3636) (1.8024, -23.2117) (1.5665, -23.0242) (1.4049, -22.9822) knots 0 0 0 1 2 2 2
  spline S143 degree 2 poles (1.4049, -22.9822) (1.2013, -22.9273) (0.7392, -22.8336) (0.5356, -22.7625) knots 0 0 0 1 2 2 2
  spline S144 degree 2 poles (0.5356, -22.7625) (0.0735, -22.6009) (-0.3272, -22.0483) (-0.3272, -21.6347) knots 0 0 0 1 2 2 2
  spline S145 degree 2 poles (-0.3272, -21.6347) (-0.3272, -21.0756) (0.6196, -20.3808) (1.3306, -20.3808) knots 0 0 0 1 2 2 2
  spline S146 degree 2 poles (1.3306, -20.3808) (1.6861, -20.3808) (2.3905, -20.5262) (2.6685, -20.649) knots 0 0 0 1 2 2 2
  line L163 (2.6685, -20.649) -> (2.6685, -21.5603)
  line L164 (2.6685, -21.5603) -> (2.5812, -21.5603)
  spline S147 degree 2 poles (2.5812, -21.5603) (2.3582, -21.3697) (1.7184, -21.1079) (1.3823, -21.1079) knots 0 0 0 1 2 2 2
  spline S148 degree 2 poles (1.3823, -21.1079) (1.2498, -21.1079) (1.043, -21.1467) (0.9266, -21.1984) knots 0 0 0 1 2 2 2
  spline S149 degree 2 poles (0.9266, -21.1984) (0.8329, -21.2404) (0.6972, -21.4084) (0.6972, -21.5119) knots 0 0 0 1 2 2 2
  spline S150 degree 2 poles (0.6972, -21.5119) (0.6972, -21.667) (0.9137, -21.8447) (1.2239, -21.9158) knots 0 0 0 1 2 2 2
  spline S151 degree 2 poles (1.2239, -21.9158) (1.4243, -21.961) (1.7959, -22.0483) (2.0092, -22.1226) knots 0 0 0 1 2 2 2
  spline S152 degree 2 poles (2.0092, -22.1226) (2.4229, -22.2745) (2.8268, -22.7786) (2.8268, -23.1923) knots 0 0 0 1 2 2 2
  spline S153 degree 2 poles (2.8268, -23.1923) (2.8268, -23.7869) (1.8929, -24.5108) (1.0979, -24.5108) knots 0 0 0 1 2 2 2
  line L165 (6.0907, -21.4311) -> (4.5751, -25.5417)
  line L166 (4.5751, -25.5417) -> (3.5668, -25.5417)
  line L167 (3.5668, -25.5417) -> (4.0225, -24.3654)
  line L168 (4.0225, -24.3654) -> (2.9205, -21.4311)
  line L169 (2.9205, -21.4311) -> (3.9029, -21.4311)
  line L170 (3.9029, -21.4311) -> (4.5363, -23.3183)
  line L171 (4.5363, -23.3183) -> (5.1277, -21.4311)
  line L172 (5.1277, -21.4311) -> (6.0907, -21.4311)
  spline S154 degree 2 poles (7.3575, -24.5205) (7.0279, -24.5205) (6.4365, -24.3751) (6.2426, -24.2781) knots 0 0 0 1 2 2 2
  line L173 (6.2426, -24.2781) -> (6.2426, -23.4864)
  line L174 (6.2426, -23.4864) -> (6.3202, -23.4864)
  spline S155 degree 2 poles (6.3202, -23.4864) (6.388, -23.5381) (6.5593, -23.6609) (6.7112, -23.7287) knots 0 0 0 1 2 2 2
  spline S156 degree 2 poles (6.7112, -23.7287) (6.8437, -23.7901) (7.1701, -23.8774) (7.364, -23.8774) knots 0 0 0 1 2 2 2
  spline S157 degree 2 poles (7.364, -23.8774) (7.5611, -23.8774) (7.8649, -23.7546) (7.8649, -23.6221) knots 0 0 0 1 2 2 2
  spline S158 degree 2 poles (7.8649, -23.6221) (7.8649, -23.5187) (7.7259, -23.4088) (7.5256, -23.3636) knots 0 0 0 1 2 2 2
  spline S159 degree 2 poles (7.5256, -23.3636) (7.4189, -23.3345) (7.0925, -23.2731) (6.9665, -23.2343) knots 0 0 0 1 2 2 2
  spline S160 degree 2 poles (6.9665, -23.2343) (6.611, -23.1244) (6.2555, -22.6946) (6.2555, -22.3424) knots 0 0 0 1 2 2 2
  spline S161 degree 2 poles (6.2555, -22.3424) (6.2555, -22.142) (6.4397, -21.7865) (6.6207, -21.6476) knots 0 0 0 1 2 2 2
  spline S162 degree 2 poles (6.6207, -21.6476) (6.7985, -21.5119) (7.3252, -21.3503) (7.6581, -21.3503) knots 0 0 0 1 2 2 2
  spline S163 degree 2 poles (7.6581, -21.3503) (7.9748, -21.3503) (8.5047, -21.4763) (8.6857, -21.5636) knots 0 0 0 1 2 2 2
  line L175 (8.6857, -21.5636) -> (8.6857, -22.3262)
  line L176 (8.6857, -22.3262) -> (8.6114, -22.3262)
  spline S164 degree 2 poles (8.6114, -22.3262) (8.5629, -22.2874) (8.3529, -22.1614) (8.2559, -22.1162) knots 0 0 0 1 2 2 2
  spline S165 degree 2 poles (8.2559, -22.1162) (8.1363, -22.0645) (7.8455, -21.9934) (7.6936, -21.9934) knots 0 0 0 1 2 2 2
  spline S166 degree 2 poles (7.6936, -21.9934) (7.49, -21.9934) (7.2089, -22.1323) (7.2089, -22.2454) knots 0 0 0 1 2 2 2
  spline S167 degree 2 poles (7.2089, -22.2454) (7.2089, -22.3488) (7.3478, -22.4652) (7.5805, -22.5233) knots 0 0 0 1 2 2 2
  spline S168 degree 2 poles (7.5805, -22.5233) (7.7001, -22.5524) (8.0135, -22.6074) (8.159, -22.6558) knots 0 0 0 1 2 2 2
  spline S169 degree 2 poles (8.159, -22.6558) (8.4821, -22.7592) (8.8182, -23.1632) (8.8182, -23.4993) knots 0 0 0 1 2 2 2
  spline S170 degree 2 poles (8.8182, -23.4993) (8.8182, -23.7093) (8.6211, -24.0939) (8.4369, -24.2232) knots 0 0 0 1 2 2 2
  spline S171 degree 2 poles (8.4369, -24.2232) (8.2462, -24.3654) (7.7227, -24.5205) (7.3575, -24.5205) knots 0 0 0 1 2 2 2
  spline S172 degree 2 poles (10.4146, -24.4979) (9.8426, -24.4979) (9.3191, -24.026) (9.3191, -23.4896) knots 0 0 0 1 2 2 2
  line L177 (9.3191, -23.4896) -> (9.3191, -22.0838)
  line L178 (9.3191, -22.0838) -> (8.9604, -22.0838)
  line L179 (8.9604, -22.0838) -> (8.9604, -21.4311)
  line L180 (8.9604, -21.4311) -> (9.3191, -21.4311)
  line L181 (9.3191, -21.4311) -> (9.3191, -20.5715)
  line L182 (9.3191, -20.5715) -> (10.2563, -20.5715)
  line L183 (10.2563, -20.5715) -> (10.2563, -21.4311)
  line L184 (10.2563, -21.4311) -> (11.1611, -21.4311)
  line L185 (11.1611, -21.4311) -> (11.1611, -22.0838)
  line L186 (11.1611, -22.0838) -> (10.2563, -22.0838)
  line L187 (10.2563, -22.0838) -> (10.2563, -23.1535)
  spline S173 degree 2 poles (10.2563, -23.1535) (10.2563, -23.3119) (10.2627, -23.5478) (10.3015, -23.6415) knots 0 0 0 1 2 2 2
  spline S174 degree 2 poles (10.3015, -23.6415) (10.3403, -23.7352) (10.531, -23.8451) (10.7119, -23.8451) knots 0 0 0 1 2 2 2
  spline S175 degree 2 poles (10.7119, -23.8451) (10.7895, -23.8451) (11.0319, -23.7804) (11.0803, -23.7546) knots 0 0 0 1 2 2 2
  line L188 (11.0803, -23.7546) -> (11.1611, -23.7546)
  line L189 (11.1611, -23.7546) -> (11.1611, -24.4138)
  spline S176 degree 2 poles (11.1611, -24.4138) (11.0092, -24.4526) (10.6667, -24.4979) (10.4146, -24.4979) knots 0 0 0 1 2 2 2
  spline S177 degree 2 poles (13.0839, -24.5205) (12.2308, -24.5205) (11.3227, -23.7061) (11.3227, -22.9531) knots 0 0 0 1 2 2 2
  spline S178 degree 2 poles (11.3227, -22.9531) (11.3227, -22.2163) (12.1694, -21.3373) (12.932, -21.3373) knots 0 0 0 1 2 2 2
  spline S179 degree 2 poles (12.932, -21.3373) (13.6204, -21.3373) (14.3184, -22.0838) (14.3184, -22.7754) knots 0 0 0 1 2 2 2
  line L190 (14.3184, -22.7754) -> (14.3184, -23.1147)
  line L191 (14.3184, -23.1147) -> (12.2599, -23.1147)
  spline S180 degree 2 poles (12.2599, -23.1147) (12.2728, -23.3248) (12.4247, -23.6027) (12.5475, -23.6867) knots 0 0 0 1 2 2 2
  spline S181 degree 2 poles (12.5475, -23.6867) (12.667, -23.7707) (12.9902, -23.8418) (13.1809, -23.8418) knots 0 0 0 1 2 2 2
  spline S182 degree 2 poles (13.1809, -23.8418) (13.3425, -23.8418) (13.6591, -23.7707) (13.7916, -23.7093) knots 0 0 0 1 2 2 2
  spline S183 degree 2 poles (13.7916, -23.7093) (13.908, -23.6609) (14.1019, -23.5413) (14.1633, -23.4961) knots 0 0 0 1 2 2 2
  line L192 (14.1633, -23.4961) -> (14.2635, -23.4961)
  line L193 (14.2635, -23.4961) -> (14.2635, -24.2716)
  spline S184 degree 2 poles (14.2635, -24.2716) (14.1471, -24.3169) (13.9597, -24.3944) (13.7916, -24.4332) knots 0 0 0 1 2 2 2
  spline S185 degree 2 poles (13.7916, -24.4332) (13.6398, -24.4752) (13.3166, -24.5205) (13.0839, -24.5205) knots 0 0 0 1 2 2 2
  spline S186 degree 2 poles (13.3942, -22.5492) (13.3877, -22.2519) (13.1259, -21.9384) (12.8577, -21.9384) knots 0 0 0 1 2 2 2
  spline S187 degree 2 poles (12.8577, -21.9384) (12.583, -21.9384) (12.2728, -22.268) (12.2566, -22.5492) knots 0 0 0 1 2 2 2
  line L194 (12.2566, -22.5492) -> (13.3942, -22.5492)
  line L195 (18.3902, -24.4397) -> (18.3902, -22.937)
  spline S188 degree 2 poles (18.3902, -22.937) (18.3902, -22.714) (18.3741, -22.4102) (18.3353, -22.3133) knots 0 0 0 1 2 2 2
  spline S189 degree 2 poles (18.3353, -22.3133) (18.2933, -22.2163) (18.1252, -22.1291) (17.9733, -22.1291) knots 0 0 0 1 2 2 2
  spline S190 degree 2 poles (17.9733, -22.1291) (17.8667, -22.1291) (17.6599, -22.2228) (17.5371, -22.3101) knots 0 0 0 1 2 2 2
  line L196 (17.5371, -22.3101) -> (17.5371, -24.4397)
  line L197 (17.5371, -24.4397) -> (16.5934, -24.4397)
  line L198 (16.5934, -24.4397) -> (16.5934, -22.937)
  spline S191 degree 2 poles (16.5934, -22.937) (16.5934, -22.7172) (16.5741, -22.4102) (16.5353, -22.3133) knots 0 0 0 1 2 2 2
  spline S192 degree 2 poles (16.5353, -22.3133) (16.4933, -22.2163) (16.3252, -22.1291) (16.1733, -22.1291) knots 0 0 0 1 2 2 2
  spline S193 degree 2 poles (16.1733, -22.1291) (16.0602, -22.1291) (15.8373, -22.2357) (15.7338, -22.3101) knots 0 0 0 1 2 2 2
  line L199 (15.7338, -22.3101) -> (15.7338, -24.4397)
  line L200 (15.7338, -24.4397) -> (14.7967, -24.4397)
  line L201 (14.7967, -24.4397) -> (14.7967, -21.4311)
  line L202 (14.7967, -21.4311) -> (15.7338, -21.4311)
  line L203 (15.7338, -21.4311) -> (15.7338, -21.7639)
  spline S194 degree 2 poles (15.7338, -21.7639) (15.9633, -21.57) (16.3737, -21.3503) (16.629, -21.3503) knots 0 0 0 1 2 2 2
  spline S195 degree 2 poles (16.629, -21.3503) (16.9037, -21.3503) (17.3238, -21.612) (17.4337, -21.8738) knots 0 0 0 1 2 2 2
  spline S196 degree 2 poles (17.4337, -21.8738) (17.7019, -21.6217) (18.1802, -21.3503) (18.4258, -21.3503) knots 0 0 0 1 2 2 2
  spline S197 degree 2 poles (18.4258, -21.3503) (18.6358, -21.3503) (18.9687, -21.4828) (19.0818, -21.6185) knots 0 0 0 1 2 2 2
  spline S198 degree 2 poles (19.0818, -21.6185) (19.2078, -21.7639) (19.3338, -22.1614) (19.3338, -22.4813) knots 0 0 0 1 2 2 2
  line L204 (19.3338, -22.4813) -> (19.3338, -24.4397)
  line L205 (19.3338, -24.4397) -> (18.3902, -24.4397)
  spline S199 degree 2 poles (20.9432, -24.5205) (20.6136, -24.5205) (20.0222, -24.3751) (19.8283, -24.2781) knots 0 0 0 1 2 2 2
  line L206 (19.8283, -24.2781) -> (19.8283, -23.4864)
  line L207 (19.8283, -23.4864) -> (19.9058, -23.4864)
  spline S200 degree 2 poles (19.9058, -23.4864) (19.9737, -23.5381) (20.145, -23.6609) (20.2969, -23.7287) knots 0 0 0 1 2 2 2
  spline S201 degree 2 poles (20.2969, -23.7287) (20.4294, -23.7901) (20.7558, -23.8774) (20.9496, -23.8774) knots 0 0 0 1 2 2 2
  spline S202 degree 2 poles (20.9496, -23.8774) (21.1468, -23.8774) (21.4505, -23.7546) (21.4505, -23.6221) knots 0 0 0 1 2 2 2
  spline S203 degree 2 poles (21.4505, -23.6221) (21.4505, -23.5187) (21.3116, -23.4088) (21.1112, -23.3636) knots 0 0 0 1 2 2 2
  spline S204 degree 2 poles (21.1112, -23.3636) (21.0046, -23.3345) (20.6782, -23.2731) (20.5522, -23.2343) knots 0 0 0 1 2 2 2
  spline S205 degree 2 poles (20.5522, -23.2343) (20.1967, -23.1244) (19.8412, -22.6946) (19.8412, -22.3424) knots 0 0 0 1 2 2 2
  spline S206 degree 2 poles (19.8412, -22.3424) (19.8412, -22.142) (20.0254, -21.7865) (20.2064, -21.6476) knots 0 0 0 1 2 2 2
  spline S207 degree 2 poles (20.2064, -21.6476) (20.3841, -21.5119) (20.9109, -21.3503) (21.2437, -21.3503) knots 0 0 0 1 2 2 2
  spline S208 degree 2 poles (21.2437, -21.3503) (21.5604, -21.3503) (22.0904, -21.4763) (22.2714, -21.5636) knots 0 0 0 1 2 2 2
  line L208 (22.2714, -21.5636) -> (22.2714, -22.3262)
  line L209 (22.2714, -22.3262) -> (22.197, -22.3262)
  spline S209 degree 2 poles (22.197, -22.3262) (22.1486, -22.2874) (21.9385, -22.1614) (21.8416, -22.1162) knots 0 0 0 1 2 2 2
  spline S210 degree 2 poles (21.8416, -22.1162) (21.722, -22.0645) (21.4312, -21.9934) (21.2793, -21.9934) knots 0 0 0 1 2 2 2
  spline S211 degree 2 poles (21.2793, -21.9934) (21.0757, -21.9934) (20.7945, -22.1323) (20.7945, -22.2454) knots 0 0 0 1 2 2 2
  spline S212 degree 2 poles (20.7945, -22.2454) (20.7945, -22.3488) (20.9335, -22.4652) (21.1662, -22.5233) knots 0 0 0 1 2 2 2
  spline S213 degree 2 poles (21.1662, -22.5233) (21.2857, -22.5524) (21.5992, -22.6074) (21.7446, -22.6558) knots 0 0 0 1 2 2 2
  spline S214 degree 2 poles (21.7446, -22.6558) (22.0678, -22.7592) (22.4039, -23.1632) (22.4039, -23.4993) knots 0 0 0 1 2 2 2
  spline S215 degree 2 poles (22.4039, -23.4993) (22.4039, -23.7093) (22.2067, -24.0939) (22.0225, -24.2232) knots 0 0 0 1 2 2 2
  spline S216 degree 2 poles (22.0225, -24.2232) (21.8319, -24.3654) (21.3084, -24.5205) (20.9432, -24.5205) knots 0 0 0 1 2 2 2
  point P0 (0, 0)
  point P1 (-28.8096, -19.625)
  point P2 (0.29, -14.0054)
  constraints: 6 midpoint, 4 end point, 2 point on line, 2 other
extrude "Extrusion7" cut sketch "Sketch6" against normal blind 1.5 contours L10 L11 L12 L13 L14 L15 | L16 L17 L18 L19 L20 L21 L22 L23 L24 L25 L26 L27 | S0 S1 S2 S3 L28 L29 S4 S5 S6 S7 S8 S9 L30 L31 L32 L33 L34 | S10 S11 S12 S13 | L35 L36 L37 L38 L39 L40 L41 S22 S23 S24 L42 | S29 S30 S31 S32 L46 L47 S33 S34 S35 S36 S37 S38 L48 L49 L50 L51 L52 | S39 S40 L53 L54 L55 S41 S42 S43 L56 S44 | L63 L64 L65 L66 | S53 S54 S55 S56 L67 L68 S57 S58 S59 S60 S61 S62 S63 S64 L69 L70 S65 S66 | S67 S68 S69 S70 | L71 L72 S79 S80 S81 L73 L74 L75 L76 L77 S82 S83 L78 | S84 L79 L80 L81 L82 L83 L84 L85 L86 L87 L88 L89 S85 S86 S87 L90 L91 S88 | L92 S89 S90 L93 L94 L95 L96 L97 S91 S92 S93 L98 | S94 S95 S96 S97 | L99 L100 L101 L102 | L103 L104 L105 L106 | S106 S107 S108 L107 L108 S109 S110 S111 S112 L109 L110 S113 S114 | L112 S117 S118 L113 L114 L115 L116 L117 S119 S120 S121 L118 | S122 S123 L119 L120 L121 L122 L123 S124 S125 | L125 L126 L127 L128 L129 L130 L131 L132 | L133 L134 L135 L136 L137 L138 L139 L140 L141 L142 | S130 S131 L143 L144 L145 S132 S133 | L149 L150 L151 L152 L153 L154 L155 L156 L157 L158 L159 L160 | S138 L161 L162 S139 S140 S141 S142 S143 S144 S145 S146 L163 L164 S147 S148 S149 S150 S151 S152 S153 | L165 L166 L167 L168 L169 L170 L171 L172 | S154 L173 L174 S155 S156 S157 S158 S159 S160 S161 S162 S163 L175 L176 S164 S165 S166 S167 S168 S169 S170 S171 | S172 L177 L178 L179 L180 L181 L182 L183 L184 L185 L186 L187 S173 S174 S175 L188 L189 S176 | S177 S178 S179 L190 L191 S180 S181 S182 S183 L192 L193 S184 S185 | L195 S188 S189 S190 L196 L197 L198 S191 S192 S193 L199 L200 L201 L202 L203 S194 S195 S196 S197 S198 L204 L205 | S199 L206 L207 S200 S201 S202 S203 S204 S205 S206 S207 S208 L208 L209 S209 S210 S211 S212 S213 S214 S215 S216
sketch "Sketch7" plane through (-21.46, -43.75, 0) normal (0, -1, 0) x (1, 0, 0)
  line L0 (0, 6) -> (43.5, 6) projected
  line L1 (0, 0) -> (0, 6) projected
  line L2 (43.5, 0) -> (43.5, 6) projected
  line L3 (0, 0) -> (43.5, 0) projected
  line L4 (15.4, 6) -> (15.4, 0)
  line L5 (43.5, 0) -> (0, 0) projected
  line L6 (28.1, 6) -> (28.1, 0)
  line L7 (15.4, 3) -> (28.1, 3) construction
  line L8 (21.75, 6) -> (21.75, 0) construction
  line L9 (0, 0) -> (43.5, 0) construction
  point P0 (21.46, 0)
  point P1 (21.75, 3)
  point P2 (28.1, 0)
  dimension "d26" = 12.7
  constraints: 8 end point, 6 midpoint, 4 point on line, 2 perpendicular
  measures "d26" distance between parallel lines of L6 L4
extrude "Extrusion8" cut sketch "Sketch7" against normal blind 8 contours L0 L6 L3 L4
body "Solid2"
